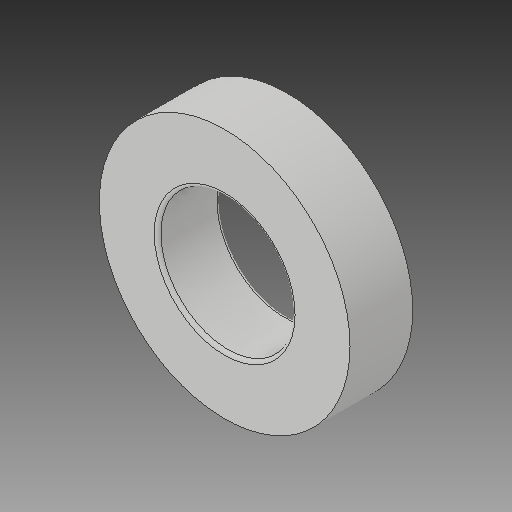
# Autodesk Inventor part: Wheel_16-30
Saved by Autodesk Inventor 2017 (Build 210142000, 142)
## iProperties
Created: 2017-03-22
Part Number: Wheel_16-30
Material: Generic
Document SubType Name: Modeling
Designer: Ali
Density: 1 g/cm^3
Appearance: Default
Author: Ali
Autodesk Inventor part; units mm, degrees
ref_plane "YZ Plane" through (0, 0, 0) normal (1, 0, 0) x (0, 1, 0)
ref_plane "XZ Plane" through (0, 0, 0) normal (0, 1, 0) x (-1, 0, 0)
ref_plane "XY Plane" through (0, 0, 0) normal (0, 0, 1) x (1, 0, 0)
sketch "Sketch1" plane through (0, 0, 0) normal (0, 0, 1) x (1, 0, 0)
  circle A0 centre (0, 0) radius 8.025
  circle A1 centre (0, 0) radius 0.3163
  circle A2 centre (0, 0) radius 15
  dimension "d0" = 16.05
  dimension "d1" = 30
  constraints: 3 centre point, 3 coincident
  measures "d0" diameter of A0
  measures "d1" diameter of A2
extrude "Extrusion1" add sketch "Sketch1" along normal blind 7.5 contours A2
fillet "Fillet1" radius 0.4 2 edges at (-8.025, 0, 7.5) (-8.025, 0, 0)
body "Solid1"
